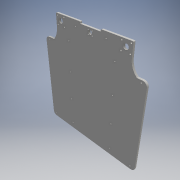
# Autodesk Inventor part: base da mesa de impressao
Saved by Autodesk Inventor 2016 (Build 200138000, 138)
## iProperties
Created: 2016-08-08
Part Number: base da mesa de impressao
Material: Generic
Document SubType Name: Modeling
Designer: Waldo
Density: 1 g/cm^3
Appearance: Default
Author: Waldo
Autodesk Inventor part; units mm, degrees
ref_plane "YZ Plane" through (0, 0, 0) normal (1, 0, 0) x (0, 1, 0)
ref_plane "XZ Plane" through (0, 0, 0) normal (0, 1, 0) x (-1, 0, 0)
ref_plane "XY Plane" through (0, 0, 0) normal (0, 0, 1) x (1, 0, 0)
sketch "Sketch1" plane through (0, 0, 0) normal (0, 1, 0) x (-1, 0, 0)
  arc A0 (32.1154, 16) -> (30.1154, 14) centre (32.1154, 14) ccw
  line L0 (30.1154, 14) -> (30.1154, 10.91)
  line L1 (30.1154, 10.91) -> (-30.1154, 10.91)
  line L2 (-30.1154, 14) -> (-30.1154, 10.91)
  arc A1 (-30.1154, 14) -> (-32.1154, 16) centre (-32.1154, 14) ccw
  line L3 (-109, 16) -> (-32.1154, 16)
  arc A2 (-109, 16) -> (-111, 14) centre (-109, 14) ccw
  line L4 (-111, 14) -> (-111, -16.0875)
  arc A3 (-127.2776, -54.7893) -> (-111, -16.0875) centre (-158.9474, -18.6953) ccw
  line L5 (-127.2776, -54.7893) -> (-140.2776, -54.7893)
  arc A4 (-140.2776, -54.7893) -> (-152.2776, -66.7893) centre (-140.2776, -66.7893) ccw
  line L6 (-152.2776, -66.7893) -> (-152.2776, -304)
  arc A5 (-152.2776, -304) -> (-140.2776, -316) centre (-140.2776, -304) ccw
  line L7 (146.9429, -316) -> (-140.2776, -316)
  arc A6 (146.9429, -316) -> (158.9429, -304) centre (146.9429, -304) ccw
  line L8 (158.9429, -66.7893) -> (158.9429, -304)
  arc A7 (158.9429, -66.7893) -> (146.9429, -54.7893) centre (146.9429, -66.7893) ccw
  line L9 (126.134, -54.7893) -> (146.9429, -54.7893)
  arc A8 (111, -16.0875) -> (126.134, -54.7893) centre (168.0523, -16.0875) ccw
  line L10 (111, 14) -> (111, -16.0875)
  arc A9 (111, 14) -> (109, 16) centre (109, 14) ccw
  line L11 (109, 16) -> (32.1154, 16)
  circle A10 centre (44.6644, 1) radius 1.5
  circle A11 centre (70.3321, -126) radius 1.5
  circle A12 centre (70.3321, -296) radius 1.5
  circle A13 centre (-44.6644, 1) radius 1.5
  circle A14 centre (-70.3321, -296) radius 1.5
  circle A15 centre (-70.3321, -211) radius 1.5
  circle A16 centre (-70.3321, -126) radius 1.5
  circle A17 centre (-70.3321, -41) radius 1.5
  circle A18 centre (-138.2776, -61) radius 1.5
  circle A19 centre (-138.2776, -306) radius 1.5
  circle A20 centre (146.7224, -306) radius 1.5
  circle A21 centre (5.6569, -5.6569) radius 1.5
  circle A22 centre (-5.6569, -5.6569) radius 1.5
  circle A23 centre (-5.6569, 5.6569) radius 1.5
  circle A24 centre (5.6569, 5.6569) radius 1.5
  circle A25 centre (83.6863, -11.3137) radius 2
  circle A26 centre (0, 0) radius 5.25
  circle A27 centre (-95, 0) radius 6.75
  circle A28 centre (95, 0) radius 6.75
  circle A29 centre (146.7224, -61) radius 1.5
  circle A30 centre (-83.6863, 11.3137) radius 2
  circle A31 centre (-106.3137, 11.3137) radius 2
  circle A32 centre (-83.6863, -11.3137) radius 2
  circle A33 centre (-106.3137, -11.3137) radius 2
  circle A34 centre (106.3137, -11.3137) radius 2
  circle A35 centre (83.6863, 11.3137) radius 2
  circle A36 centre (70.3321, -211) radius 1.5
  circle A37 centre (70.3321, -41) radius 1.5
  circle A38 centre (106.3137, 11.3137) radius 2
  point P0 (0, 0)
  constraints: 39 centre point, 32 equal radius, 24 end point, 21 tangent, 20 point on circle, 5 parallel, 4 perpendicular
extrude "Extrusion1" add sketch "Sketch1" along normal blind 6
body "Solid1"
